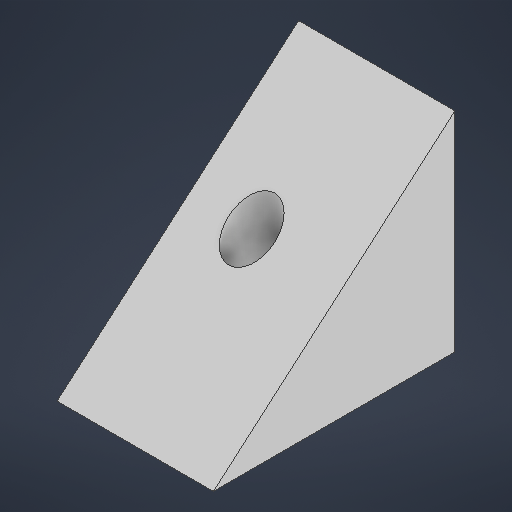
# Autodesk Inventor part: Intake Angle Mount
Saved by Autodesk Inventor 2025 (Build 290162000, 162)
## iProperties
Created: 2025-02-17
Part Number: Intake Angle Mount
Material: Generic
Document SubType Name: Modeling
Designer: Juan
Density: 1 g/cm^3
Appearance: Default
Author: Juan
Autodesk Inventor part; units mm, degrees
ref_plane "YZ Plane" through (0, 0, 0) normal (1, 0, 0) x (0, 1, 0)
ref_plane "XZ Plane" through (0, 0, 0) normal (0, 1, 0) x (-1, 0, 0)
ref_plane "XY Plane" through (0, 0, 0) normal (0, 0, 1) x (1, 0, 0)
sketch "Sketch1" plane through (0, 0, 0) normal (1, 0, 0) x (0, 1, 0)
  line L0 (26.0516, -1.632) -> (-7.8592, 37.6025)
  line L1 (30.2039, -6.4362) -> (26.0516, -1.632)
  line L2 (-5.4571, 39.6786) -> (28.4537, 0.4442)
  circle A0 centre (-29.6949, -7.0287) radius 2.1844
  circle A1 centre (-29.6949, -32.4287) radius 2.1844
  line L3 (-23.764, -36.7467) -> (-23.764, 23.7053)
  circle A2 centre (-29.6949, 18.3713) radius 2.1844
  line L4 (-23.764, 18.3713) -> (-21.7574, 18.3713)
  line L5 (-21.7574, 18.3713) -> (-2.8344, 18.3713)
  line L6 (-2.8344, 18.3713) -> (-2.8344, 12.0213)
  line L7 (-2.8344, 12.0213) -> (-2.8344, 24.7213)
  line L8 (-2.8344, 24.7213) -> (3.2741, 24.7213)
  line L9 (-2.8344, 12.0213) -> (14.2509, 12.0213)
  line L10 (-2.8344, 18.3713) -> (-2.8344, 13.6088)
  line L11 (-2.8344, 13.6088) -> (-2.8344, 23.1338)
  line L12 (-2.8344, 23.1338) -> (4.6462, 23.1338)
  line L13 (-2.8344, 13.6088) -> (12.8788, 13.6088)
  line L14 (-29.6949, 18.3713) -> (-29.6949, 31.3507)
  line L15 (-29.6949, 31.3507) -> (-2.4557, 31.3507)
  line L16 (-29.6949, 31.3507) -> (-29.6949, 34.5257)
  line L17 (-29.6949, 34.5257) -> (-5.1999, 34.5257)
  line L18 (-29.6949, 18.3713) -> (-29.6949, 5.2395)
  line L19 (-29.6949, 5.2395) -> (20.1125, 5.2395)
  line L20 (-29.6949, 5.2395) -> (-29.6949, 2.0645)
  line L21 (-29.6949, 2.0645) -> (22.8567, 2.0645)
  point P0 (0, 0)
  point P1 (-23.764, 2.0645)
  point P2 (-23.764, 5.2395)
  dimension "d0" = 2.0066
  dimension "d3" = 12.7
  dimension "d4" = 4.7625
  dimension "d5" = 9.525
  dimension "d6" = 12.9794
  dimension "d7" = 3.175
  dimension "d8" = 13.1318
  dimension "d9" = 3.175
  constraints: 42 end point, 5 horizontal, 5 point on line, 5 vertical, 4 perpendicular, 3 centre point, 11 other
  measures "d0" distance of L4.start L4.end
  measures "d3" distance of L6.end L7.end
  measures "d4" distance of L5.end L10.end
  measures "d5" distance of L10.end L11.end
  measures "d6" distance of L14.start L14.end
  measures "d7" distance of L14.end L16.end
  measures "d8" distance of L14.start L18.end
  measures "d9" distance of L18.end L20.end
extrude "Extrusion2" add sketch "Sketch1" against normal blind 15.875 contours L13 L6 L7 L12 L0
sketch "Sketch2" plane through (0, -2.8344, 13.6088) normal (0, -1, 0) x (1, 0, 0)
  line L0 (0, 9.525) -> (0, 0) projected
  line L1 (0, 9.525) -> (-15.875, 9.525) projected
  line L2 (-15.875, 0) -> (-15.875, 9.525) projected
  line L3 (0, 0) -> (-15.875, 0) projected
  line L4 (0, 4.7625) -> (-9.525, 4.7625)
  circle A0 centre (-9.525, 4.7625) radius 2.3241
  point P0 (0, -13.6088)
  dimension "d14" = 9.525
  dimension "d15" = 4.6482
  constraints: 2 end point, 1 centre point, 1 coincident, 1 horizontal, 1 midpoint
  measures "d14" distance of L4.start L4.end
  measures "d15" diameter of A0
extrude "Extrusion3" cut sketch "Sketch2" against normal through all contours A0
move faces "Move1" translate (0, 0, 36.5252) faces at (-5.2917, 2.1527, 23.1338)
move faces "Move2" translate (0, 0, -6.35) faces at (-5.2917, 2.4033, 13.6088)
sketch "Sketch3" plane through (-15.875, 0, 0) normal (-1, 0, 0) x (0, 0, 1)
  line L0 (7.2588, -2.8344) -> (31.7888, -2.8344) projected
  circle A0 centre (7.2588, -2.8344) radius 9.525
  circle A1 centre (3.0867, -11.3971) radius 21.1023
  point P0 (0, 0)
  dimension "d24" = 19.05
  constraints: 1 centre point, 3 other
extrude "Extrusion5" cut sketch "Sketch3" against normal blind 3.175 contours A0 | A1
fillet "Fillet2" radius 3.175 2 edges at (-12.7, 5.0645, 16.2899) (-15.875, 5.0645, 16.2899)
body "Solid2"
